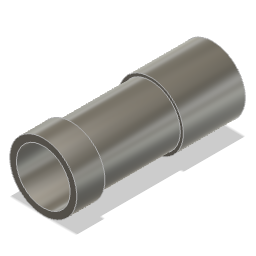
SFMJoiner (Autodesk Fusion 360 design; units mm, degrees)
Autodesk Fusion 360 part; units mm, degrees
note: some values were not read from the file. Set by a fixed rule: which sketch regions a step uses.
sketch "Sketch1" plane through (0, 0, 0) normal (1, 0, 0) x (0, 0, -1)
  line L0 (-41.9028, 11) -> (-71.5, 11)
  line L1 (-82, 11) -> (-82, 12.5)
  line L2 (-82, 12.5) -> (-71.5, 12.5)
  line L3 (-71.5, 12.5) -> (-71.5, 11)
  line L4 (-71.5, 11) -> (-41.9028, 11)
  line L5 (-41, 11) -> (-41, 10)
  line L6 (-41, 10) -> (-82, 10)
  line L7 (-82, 10) -> (-82, 11)
  line L8 (-21.273, 11.3453) -> (-41, 11.3453)
  line L9 (-41, 11.3453) -> (-41, 11)
  line L10 (-21.273, 12.1453) -> (-41.9028, 12.1453)
  line L11 (-41.9028, 12.1453) -> (-41.9028, 11)
  line L12 (-20.7884, 12.1453) -> (-21.273, 12.1453)
  line L13 (-20.7884, 12.1453) -> (-18.8, 12.1453)
  line L14 (-18.8, 12.1453) -> (-18.8, 11.3453)
  line L15 (-21.1992, 11.3453) -> (-21.273, 11.3453)
  line L16 (-21.1992, 11.3453) -> (-21.0412, 11.2127)
  line L17 (-18.8, 11.3453) -> (-18.8139, 11.3287)
  line L18 (-21.0412, 11.2127) -> (-18.8139, 11.3287)
  point P0 (-20.7884, 10.9915)
  dimension "d1" = 1.5
  dimension "d2" = 10.5
  dimension "d3" = 0.8
  dimension "d4" = 0.6
  constraint horizontal L0
  constraint perpendicular L0 L1
  constraint perpendicular L1 L2
  constraint perpendicular L0 L3
  constraint horizontal L4
  constraint vertical L5
  constraint horizontal L6
  constraint vertical L7
  constraint perpendicular L5 L8
  constraint perpendicular L0 L9
  constraint perpendicular L4 L11
  constraint parallel L12 L13
  constraint perpendicular L12 L14
  constraint perpendicular L16 L17
  measures "d1" distance of L1.start L1.end
  measures "d2" distance of L1.end L2.end
  measures "d3" distance of L8.start L10.start
  measures "d4" distance of L8.start P0
revolve "Revolve1" add sketch "Sketch1" angle 360 about axis through (0, 0, 1.75) along (0, 0, 1)
